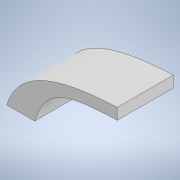
# Autodesk Inventor part: zweef
Saved by Autodesk Inventor 2021 (Build 250183000, 183)
## iProperties
Created: 2023-10-02
Part Number: zweef
Material: Generic
Document SubType Name: Modeling
Designer: Elias
Density: 1 g/cm^3
Appearance: Default
Author: Elias
Autodesk Inventor part; units mm, degrees
ref_plane "YZ Plane" through (0, 0, 0) normal (1, 0, 0) x (0, 1, 0)
ref_plane "XZ Plane" through (0, 0, 0) normal (0, 1, 0) x (-1, 0, 0)
ref_plane "XY Plane" through (0, 0, 0) normal (0, 0, 1) x (1, 0, 0)
sketch "Sketch1" plane through (0, 0, 0) normal (0, 0, 1) x (1, 0, 0)
  line L0 (0, 0) -> (5, 0)
  line L1 (0, 0) -> (2.0374, 6.5) construction
  line L2 (2.0374, 6.5) -> (8.5572, 9) construction
  line L3 (8.5572, 9) -> (19.763, 9.5) construction
  spline S0 degree 3 poles (0, 0) (2.0374, 6.5) (8.5572, 9) (19.763, 9.5) knots 1 1 1 1 2 2 2 2
  line L4 (5, 0) -> (7.0374, 6.5) construction
  line L5 (7.0374, 6.5) -> (10.843, 7.0977) construction
  line L6 (10.843, 7.0977) -> (19.5421, 7.4957) construction
  spline S1 degree 3 poles (5, 0) (7.0374, 6.5) (10.843, 7.0977) (19.5421, 7.4957) knots 1 1 1 1 2 2 2 2
  line L7 (19.763, 9.5) -> (19.763, 7.4957)
  line L8 (19.763, 7.4957) -> (19.5421, 7.4957)
  dimension "d0" = 5
  dimension "d1" = 6.5
  dimension "d3" = 9.5
  dimension "d4" = 5
  constraints: 6 end point, 1 horizontal, 1 perpendicular, 1 vertical, 6 other
  measures "d0" distance of L0.start L0.end
  measures "d1" distance from line of L0 L1.end
  measures "d3" distance from line of L0 L3.end
  measures "d4" distance of L1.end L4.end
extrude "Extrusion1" add sketch "Sketch1" along normal blind 10
body "Solid1"
